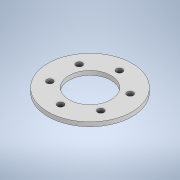
# Autodesk Inventor part: btnring
Saved by Autodesk Inventor 2022 (Build 260153000, 153)
## iProperties
Created: 2025-06-26
Part Number: btnring
Material: Типовые
Document SubType Name: Modeling
Designer: korsh624
Density: 1 g/cm^3
Appearance: По умолчанию
Author: korsh624
Autodesk Inventor part; units mm, degrees
ref_plane "YZ Plane" through (0, 0, 0) normal (1, 0, 0) x (0, 1, 0)
ref_plane "XZ Plane" through (0, 0, 0) normal (0, 1, 0) x (-1, 0, 0)
ref_plane "XY Plane" through (0, 0, 0) normal (0, 0, 1) x (1, 0, 0)
sketch "Эскиз1" plane through (0, 0, 0) normal (0, 1, 0) x (-1, 0, 0)
  circle A0 centre (0, 0) radius 20
  circle A1 centre (0, 0) radius 10
  circle A2 centre (0, -14) radius 1.5
  circle A3 centre (12.1244, -7) radius 1.5
  circle A4 centre (12.1244, 7) radius 1.5
  circle A5 centre (0, 14) radius 1.5
  circle A6 centre (-12.1244, 7) radius 1.5
  circle A7 centre (-12.1244, -7) radius 1.5
  dimension "d0" = 40
  dimension "d1" = 20
  dimension "d2" = 14
  dimension "d3" = 3
  dimension "d6" = 360
  constraints: 8 centre point, 2 coincident, 13 other
  measures "d0" diameter of A0
  measures "d1" diameter of A1
  measures "d2" distance of A2.centre point (0, 0)
  measures "d3" diameter of A2
extrude "Выдавливание1" add sketch "Эскиз1" along normal blind 2
